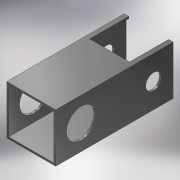
# Autodesk Inventor part: pipe_square_back
Saved by Autodesk Inventor 2018.2 (Build 222227000, 227)
## iProperties
Created: 2017-12-11
Part Number: pipe_square_back
Material: 鉄、可鍛鉄
Document SubType Name: Modeling
Designer: kuwano
Density: 7.15 g/cm^3
Appearance: 半つや出し
Author: kuwano
Autodesk Inventor part; units mm, degrees
ref_plane "YZ Plane" through (0, 0, 0) normal (1, 0, 0) x (0, 1, 0)
ref_plane "XZ Plane" through (0, 0, 0) normal (0, 1, 0) x (-1, 0, 0)
ref_plane "XY Plane" through (0, 0, 0) normal (0, 0, 1) x (1, 0, 0)
sketch "スケッチ1" plane through (0, 0, 0) normal (0, 1, 0) x (-1, 0, 0)
  line L0 (12.5, 12.5) -> (-12.5, 12.5)
  line L1 (-12.5, 12.5) -> (-12.5, -12.5)
  line L2 (-12.5, -12.5) -> (12.5, -12.5)
  line L3 (12.5, -12.5) -> (12.5, 12.5)
  line L4 (12.5, 12.5) -> (-12.5, -12.5) construction
  line L5 (-12.5, 12.5) -> (12.5, -12.5) construction
  point P0 (0, 0)
  dimension "d0" = 25
  dimension "d1" = 25
  constraints: 12 end point, 2 midpoint, 2 parallel, 1 horizontal, 1 perpendicular
  measures "d0" distance of L0.start L0.end
  measures "d1" distance of L2.end L0.start
extrude "押し出し1" add sketch "スケッチ1" along normal blind 60
shell "シェル1" thickness 1 removed faces 2 at (4.1667, 60, -4.1667) at (4.1667, 0, -4.1667)
sketch "スケッチ2" plane through (12.5, 0, 12.5) normal (1, 0, 0) x (0, 0, -1)
  circle A0 centre (12.5, 13) radius 7.5
  line L0 (0, 0) -> (25, 0) projected
  point P0 (12.5, 0)
  dimension "d5" = 13
  dimension "d6" = 15
  constraints: 1 centre point
  measures "d5" distance from line of L0 A0.centre
  measures "d6" diameter of A0
extrude "押し出し2" cut sketch "スケッチ2" against normal through all
sketch "スケッチ3" plane through (-12.5, 0, 12.5) normal (0, 0, 1) x (1, 0, 0)
  line L0 (0, 60) -> (25, 60) projected
  line L1 (2.3, 60) -> (22.7, 60)
  line L2 (22.7, 60) -> (22.7, 40)
  line L3 (22.7, 40) -> (2.3, 40)
  line L4 (2.3, 40) -> (2.3, 60)
  line L5 (0, 0) -> (0, 60) projected
  line L6 (25, 0) -> (25, 60) projected
  point P0 (12.5, 0)
  dimension "d9" = 2.3
  dimension "d10" = 2.3
  dimension "d11" = 20
  constraints: 8 end point, 2 parallel, 1 horizontal, 1 perpendicular, 1 point on line
  measures "d9" distance between parallel lines of L5 L4
  measures "d10" distance between parallel lines of L6 L2
  measures "d11" distance of L1.end L2.end
extrude "押し出し3" cut sketch "スケッチ3" against normal through all
sketch "スケッチ4" plane through (12.5, 0, 12.5) normal (1, 0, 0) x (0, 0, -1)
  circle A0 centre (12.5, 50) radius 4
  line L0 (0, 60) -> (25, 60) projected
  point P0 (12.5, 0)
  dimension "d14" = 8
  dimension "d15" = 10
  constraints: 1 centre point
  measures "d14" diameter of A0
  measures "d15" distance from line of L0 A0.centre
extrude "押し出し4" cut sketch "スケッチ4" against normal through all
equation "\"d1\" = d0"
equation "\"d10\" = d9"
